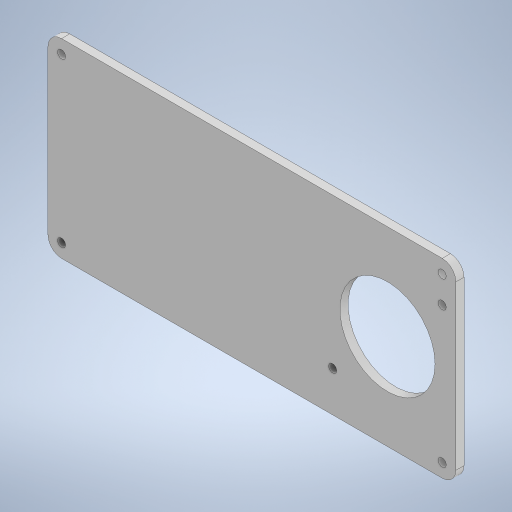
# Autodesk Inventor part: Charger ShroudPlate - EthanMockup
Saved by Autodesk Inventor 2023 (Build 270158000, 158)
## iProperties
Created: 2023-01-17
Part Number: Charger ShroudPlate - EthanMockup
Material: Generic
Document SubType Name: Modeling
Designer: ethan
Density: 1 g/cm^3
Appearance: Default
Author: ethan
Autodesk Inventor part; units mm, degrees
ref_plane "YZ Plane" through (0, 0, 0) normal (1, 0, 0) x (0, 1, 0)
ref_plane "XZ Plane" through (0, 0, 0) normal (0, 1, 0) x (-1, 0, 0)
ref_plane "XY Plane" through (0, 0, 0) normal (0, 0, 1) x (1, 0, 0)
sketch "Sketch1" plane through (0, 0, 0) normal (0, 0, 1) x (1, 0, 0)
  line L0 (0, 0) -> (150, 0)
  line L1 (150, 0) -> (150, 70)
  line L2 (150, 70) -> (0, 70)
  line L3 (0, 70) -> (0, 0)
  line L4 (5, 65) -> (145, 65) construction
  line L5 (145, 65) -> (145, 5) construction
  line L6 (145, 5) -> (5, 5) construction
  line L7 (5, 5) -> (5, 65) construction
  circle A0 centre (5, 65) radius 1.5
  circle A1 centre (5, 5) radius 1.5
  circle A2 centre (145, 5) radius 1.5
  circle A3 centre (145, 65) radius 1.5
  line L8 (104.6949, 55.1525) -> (145, 55.1525) construction
  line L9 (145, 55.1525) -> (145, 14.8475) construction
  line L10 (145, 14.8475) -> (104.6949, 14.8475) construction
  line L11 (104.6949, 14.8475) -> (104.6949, 55.1525) construction
  circle A4 centre (104.6949, 14.8475) radius 1.5
  circle A5 centre (145, 55.1525) radius 1.5
  line L12 (104.6949, 14.8475) -> (145, 55.1525) construction
  circle A6 centre (124.8475, 35) radius 17.5
  line L13 (146.5, 56.6525) -> (103.1949, 56.6525) construction
  line L14 (103.1949, 56.6525) -> (103.1949, 13.3475) construction
  line L15 (103.1949, 13.3475) -> (146.5, 13.3475) construction
  line L16 (146.5, 13.3475) -> (146.5, 56.6525) construction
  line L17 (0, 56.6525) -> (0, 58.6525)
  line L18 (103.1949, 56.6525) -> (103.1949, 35.6525) construction
  dimension "d0" = 150
  dimension "d1" = 70
  dimension "d2" = 5
  dimension "d3" = 5
  dimension "d4" = 60
  dimension "d5" = 140
  dimension "d6" = 3
  dimension "d7" = 3
  dimension "d8" = 3
  dimension "d9" = 3
  dimension "d13" = 40.3051
  dimension "d14" = 40.3051
  dimension "d15" = 3
  dimension "d16" = 3
  dimension "d17" = 14.8475
  dimension "d18" = 35
  constraints: 38 end point, 8 parallel, 7 centre point, 6 coincident, 4 horizontal, 4 perpendicular, 4 tangent, 2 point on line, 1 collinear, 1 midpoint
  measures "d0" distance of L2.end L1.end
  measures "d1" distance of L1.end L0.end
  measures "d2" distance between parallel lines of L2 L4
  measures "d3" distance between parallel lines of L3 L7
  measures "d4" distance of L4.end L5.end
  measures "d5" distance of L4.start L4.end
  measures "d6" diameter of A0
  measures "d7" diameter of A1
  measures "d8" diameter of A2
  measures "d9" diameter of A3
  measures "d13" distance of L10.end L8.start
  measures "d14" distance of L8.start L8.end
  measures "d15" diameter of A4
  measures "d16" diameter of A5
  measures "d17" distance between parallel lines of L2 L8
  measures "d18" diameter of A6
extrude "Extrusion1" add sketch "Sketch1" along normal blind 3
fillet "Fillet1" radius 5 4 edges at (0, 70, 1.5) (0, 0, 1.5) (150, 0, 1.5) (150, 70, 1.5)
equation "\"d14\" = d13"
equation "\"d17\" = -0.5 * d13 + 0.5 * d1"
body "Solid1"
